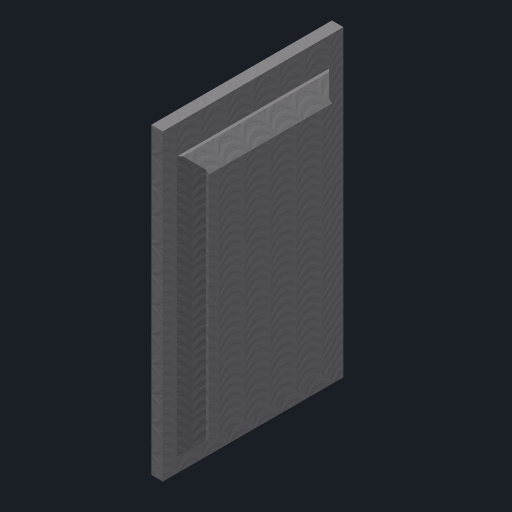
# Autodesk Inventor part: DIMENSIONES_PANTALLA
Saved by Autodesk Inventor 2024.3 (Build 283343000, 343)
## iProperties
Created: 2024-05-12
Part Number: DIMENSIONES_PANTALLA
Material: Steel, Mild, Welded
Document SubType Name: Modeling
Designer: Niler
Density: 7.85 g/cm^3
Appearance: Weld - Steel Mild
Author: Niler
Autodesk Inventor part; units mm, degrees
ref_plane "YZ Plane" through (0, 0, 0) normal (1, 0, 0) x (0, 1, 0)
ref_plane "XZ Plane" through (0, 0, 0) normal (0, 1, 0) x (-1, 0, 0)
ref_plane "XY Plane" through (0, 0, 0) normal (0, 0, 1) x (1, 0, 0)
sketch "Sketch1" plane through (0, 0, 0) normal (1, 0, 0) x (0, 1, 0)
  line L0 (-243.5, 137) -> (243.5, 137)
  line L1 (243.5, 137) -> (243.5, -137)
  line L2 (243.5, -137) -> (-243.5, -137)
  line L3 (-243.5, -137) -> (-243.5, 137)
  line L4 (-243.5, 137) -> (243.5, -137) construction
  line L5 (243.5, 137) -> (-243.5, -137) construction
  line L6 (263.5, -157) -> (263.5, 157)
  line L7 (263.5, 157) -> (-263.5, 157)
  line L8 (-263.5, 157) -> (-263.5, -157)
  line L9 (-263.5, -157) -> (263.5, -157)
  point P0 (0, 0)
  dimension "d0" = 487
  dimension "d1" = 274
  dimension "d2" = 20
  constraints: 20 end point, 4 parallel, 2 midpoint, 2 perpendicular, 1 horizontal, 3 other
  measures "d0" distance of L1.end L2.end
  measures "d1" distance of L0.end L1.end
  measures "d2" distance between parallel lines of L1 L6
extrude "Extrusion1" add sketch "Sketch1" along normal blind 20 contours L0 L1 L2 L3 | L9 L8 L7 L6
extrude "Extrusion2" cut sketch "Sketch1" along normal blind 2 contours L0 L1 L2 L3
sketch "Sketch2" plane through (20, 0, 0) normal (1, 0, 0) x (0, 0, -1)
  line L0 (-157, 263.5) -> (-157, -263.5) projected
  line L1 (-157, -263.5) -> (157, -263.5) projected
  line L2 (157, -263.5) -> (157, 263.5) projected
  line L3 (157, 263.5) -> (-157, 263.5) projected
  line L4 (-107, 213.5) -> (-107, -213.5)
  line L5 (-107, -213.5) -> (107, -213.5)
  line L6 (107, -213.5) -> (107, 213.5)
  line L7 (107, 213.5) -> (-107, 213.5)
  point P0 (0, 0)
  dimension "d7" = 50
  constraints: 8 end point, 3 other
  measures "d7" distance between parallel lines of L3 L7
extrude "Extrusion3" add sketch "Sketch2" along normal blind 30 contours L7 L6 L5 L4
chamfer "Chamfer1" distance 25 angle 45 4 edges at (20, 0, -107) (50, 213.5, 0) (20, 0, 107) (20, -213.5, 0)
body "Solid1"
